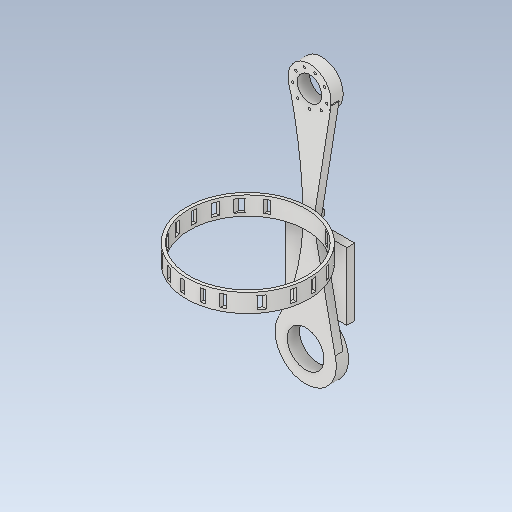
# Autodesk Inventor part: ES101_Project_Thigh support
Saved by Autodesk Inventor 2021 (Build 250183000, 183)
## iProperties
Created: 2021-03-10
Part Number: ES101_Project_Thigh support
Material: PPS Plastic
Document SubType Name: Modeling
Designer: lenovo
Density: 1.637 g/cm^3
Appearance: Smooth - White
Author: lenovo
Autodesk Inventor part; units mm, degrees
note: some values were not read from the file. Chosen so that the rebuilt part matches the saved one: second side of "Extrusion2"; second side of "Extrusion3".
ref_plane "YZ Plane" through (0, 0, 0) normal (1, 0, 0) x (0, 1, 0)
ref_plane "XY Plane" through (0, 0, 0) normal (0, 0, 1) x (1, 0, 0)
sketch "Sketch1" plane through (0, 0, 0) normal (0, 0, 1) x (1, 0, 0)
  arc A0 (-33.3712, 172.0844) -> (35.1489, 174.9362) centre (0.5971, 180.5198) ccw
  arc A1 (-50.7972, -166.0649) -> (-10.4253, -3.0182) centre (-368.5147, -0.8734) ccw
  line L0 (6.4335, -2.7585) -> (42.5482, -179.0984)
  arc A2 (42.5482, -179.0984) -> (-50.7972, -166.0649) centre (-6.4351, -189.1302) ccw
  arc A3 (-10.4253, -3.0182) -> (-33.3712, 172.0844) centre (-792.6654, -16.4703) ccw
  line L1 (6.4335, -2.7585) -> (35.1489, 174.9362)
  point P0 (0, 0)
  point P1 (-4.1446, -190.5357)
  point P2 (45.8554, -190.5357)
  dimension "d9" = 70
  dimension "d12" = 180
  dimension "d13" = 180
  dimension "d14" = 50
  constraints: 8 point on circle, 4 centre point, 4 end point, 4 tangent, 3 coincident
  measures "d9" diameter of A0
  measures "d12" distance of L0.start L0.end
  measures "d13" distance of L0.start L1.end
  measures "d14" radius of A2
extrude "Extrusion1" add sketch "Sketch1" along normal blind 13
sketch "Sketch2" plane through (0, 0, 13) normal (0, 0, 1) x (1, 0, 0)
  circle A0 centre (-6.3508, -188.8118) radius 50
  circle A1 centre (-6.3508, -188.8118) radius 30
  circle A2 centre (0, 180.6568) radius 35
  circle A3 centre (0, 180.6568) radius 20
  point P0 (0, 0)
  constraints: 4 centre point, 2 coincident
extrude "Extrusion2" add sketch "Sketch2" against normal blind 20 contours A0
sketch "Sketch3" plane through (0, 0, 13) normal (0, 0, 1) x (1, 0, 0)
  circle A0 centre (0, 182.0197) radius 35
  circle A1 centre (0, 182.0197) radius 20
  point P0 (0, 0)
  constraints: 2 centre point, 1 coincident
extrude "Extrusion3" add sketch "Sketch3" against normal blind 20
sketch "Sketch4" plane through (0, 0, 0) normal (0, 0, -1) x (-1, 0, 0)
  line L0 (-47.7429, -25.3634) -> (52.2571, -25.3634)
  line L1 (52.2571, -25.3634) -> (52.2571, -135.3634)
  line L2 (52.2571, -135.3634) -> (-47.7429, -135.3634)
  line L3 (-47.7429, -135.3634) -> (-47.7429, -25.3634)
  point P0 (0, 0)
  dimension "d32" = 100
  dimension "d33" = 110
  constraints: 8 end point, 2 parallel, 1 horizontal, 1 perpendicular
  measures "d32" distance of L1.end L2.end
  measures "d33" distance of L0.end L1.end
extrude "Extrusion4" add sketch "Sketch4" along normal blind 13
sketch "Sketch5" plane through (0, 0, 0) normal (0, 0, -1) x (-1, 0, 0)
  circle A0 centre (1.6929, -2.3398) radius 7
  point P0 (0, 0)
  constraints: 1 centre point
extrude "Extrusion5" add sketch "Sketch5" along normal blind 7
sketch "Sketch6" plane through (-1.6929, -2.3398, -7) normal (0, 0, -1) x (-1, 0, 0)
  circle A0 centre (0, 0) radius 7 projected
  circle A1 centre (0, 0) radius 5
  point P0 (-1.6929, 2.3398)
  dimension "d39" = 10
  constraints: 1 centre point, 1 coincident
  measures "d39" diameter of A1
extrude "Extrusion6" add sketch "Sketch6" along normal blind 2 contours A1
sketch "Sketch7" plane through (0, 0, 13) normal (0, 0, 1) x (1, 0, 0)
  point P0 (0, 0)
sketch "Sketch8" plane through (0, 0, 0) normal (0, 1, 0) x (-1, 0, 0)
  circle A0 centre (0, 113.7823) radius 100
  point P0 (0, 0)
  dimension "d88" = 200
  constraints: 1 centre point
  measures "d88" diameter of A0
extrude "Extrusion7" add sketch "Sketch8" along normal mid plane 30 separate body
sketch "Sketch9" plane through (0, 15, 113.7823) normal (0, 1, 0) x (1, 0, 0)
  circle A0 centre (0, 0) radius 95
  point P0 (0, 113.7823)
  dimension "d45" = 190
  constraints: 1 centre point
  measures "d45" diameter of A0
extrude "Extrusion8" cut sketch "Sketch9" against normal blind 30 bodies 2
sketch "Sketch10" plane through (0, 0, 13) normal (0, 0, 1) x (1, 0, 0)
  circle A0 centre (0, 177.9274) radius 34.5248
  point P0 (0, 0)
  constraints: 1 centre point
extrude "Extrusion9" add sketch "Sketch10" against normal blind 13 bodies 1
sketch "Sketch11" plane through (0, 182.0197, 0) normal (0, 0, -1) x (-1, 0, 0)
  circle A0 centre (0, 0) radius 20
  point P0 (0, -182.0197)
  constraints: 1 centre point
extrude "Extrusion10" cut sketch "Sketch11" against normal blind 13 bodies 1
sketch "Sketch12" plane through (0, 0, 13) normal (0, 0, 1) x (1, 0, 0)
  circle A0 centre (0, 153.4937) radius 2
  circle A1 centre (-19.2305, 158.9881) radius 2
  circle A2 centre (-27.7702, 177.0733) radius 2
  circle A3 centre (-22.2758, 196.3038) radius 2
  circle A4 centre (24.2555, 196.3038) radius 2
  circle A5 centre (28.2555, 175.0733) radius 2
  circle A6 centre (19.1953, 160.9881) radius 2
  circle A7 centre (-8.7701, 208.0286) radius 2
  circle A8 centre (9.0493, 208.0286) radius 2
  point P0 (0, 0)
  dimension "d54" = 4
  dimension "d67" = 4
  dimension "d68" = 4
  dimension "d69" = 4
  constraints: 9 centre point
  measures "d54" diameter of A0
  measures "d67" diameter of A6
  measures "d68" diameter of A7
  measures "d69" diameter of A8
extrude "Extrusion11" cut sketch "Sketch12" against normal blind 20 bodies 1
sketch "Sketch13" plane through (0, 0, 0) normal (1, 0, 0) x (0, 1, 0)
  point P0 (0, 0)
sketch "Sketch14" plane through (0, 0, 13) normal (0, 0, 1) x (1, 0, 0)
  point P0 (0, 0)
sketch "Sketch15" plane through (0, 0, 0) normal (1, 0, 0) x (0, 1, 0)
  point P0 (0, 0)
ref_plane "Work Plane1" through (0, 0, 0) normal (0, 1, 0) x (-1, 0, 0)
sketch "Sketch16" plane through (0, 0, 0) normal (0, 1, 0) x (-1, 0, 0)
  line L0 (32.5367, 18.2576) -> (29.6883, 18.2576)
  line L1 (29.6883, 18.2576) -> (29.6883, 28.4518)
  line L2 (29.6883, 28.4518) -> (32.5367, 28.4518)
  line L3 (32.5367, 28.4518) -> (32.5367, 18.2576)
  line L4 (12.3378, 34.8063) -> (36.3483, 52.7924)
  line L5 (36.3483, 52.7924) -> (49.6954, 79.6597)
  line L6 (49.6954, 79.6597) -> (51.0134, 109.6307)
  line L7 (51.0134, 109.6307) -> (41.4291, 138.0586)
  line L8 (41.4291, 138.0586) -> (20.4475, 159.5009)
  line L9 (20.4475, 159.5009) -> (-7.3084, 170.8857)
  line L10 (-7.3084, 170.8857) -> (-37.3084, 170.8857)
  line L11 (-37.3084, 170.8857) -> (-63.9806, 157.1528)
  line L12 (-63.9806, 157.1528) -> (-83.8606, 134.6853)
  line L13 (-83.8606, 134.6853) -> (-92.5467, 105.9703)
  line L14 (-92.5467, 105.9703) -> (-89.9607, 76.082)
  line L15 (-89.9607, 76.082) -> (-73.9206, 50.7302)
  line L16 (-73.9206, 50.7302) -> (-48.4956, 34.8063)
  line L17 (38.6924, 42.1786) -> (34.0041, 42.1786)
  line L18 (34.0041, 42.1786) -> (34.0041, 63.4061)
  line L19 (34.0041, 63.4061) -> (38.6924, 63.4061)
  line L20 (38.6924, 63.4061) -> (38.6924, 42.1786)
  line L21 (38.6924, 42.1786) -> (34.0041, 63.4061) construction
  line L22 (34.0041, 42.1786) -> (38.6924, 63.4061) construction
  line L23 (53.1695, 77.9338) -> (46.2212, 77.9338)
  line L24 (46.2212, 77.9338) -> (46.2212, 81.3856)
  line L25 (46.2212, 81.3856) -> (53.1695, 81.3856)
  line L26 (53.1695, 81.3856) -> (53.1695, 77.9338)
  line L27 (53.1695, 77.9338) -> (46.2212, 81.3856) construction
  line L28 (46.2212, 77.9338) -> (53.1695, 81.3856) construction
  line L29 (55.8056, 106.9834) -> (46.2212, 106.9834)
  line L30 (46.2212, 106.9834) -> (46.2212, 112.2781)
  line L31 (46.2212, 112.2781) -> (55.8056, 112.2781)
  line L32 (55.8056, 112.2781) -> (55.8056, 106.9834)
  line L33 (55.8056, 106.9834) -> (46.2212, 112.2781) construction
  line L34 (46.2212, 106.9834) -> (55.8056, 112.2781) construction
  line L35 (49.7019, 140.8477) -> (33.1562, 140.8477)
  line L36 (33.1562, 140.8477) -> (33.1562, 135.2694)
  line L37 (33.1562, 135.2694) -> (49.7019, 135.2694)
  line L38 (49.7019, 135.2694) -> (49.7019, 140.8477)
  line L39 (49.7019, 140.8477) -> (33.1562, 135.2694) construction
  line L40 (33.1562, 140.8477) -> (49.7019, 135.2694) construction
  line L41 (23.199, 166.209) -> (17.696, 166.209)
  line L42 (17.696, 166.209) -> (17.696, 152.7928)
  line L43 (17.696, 152.7928) -> (23.199, 152.7928)
  line L44 (23.199, 152.7928) -> (23.199, 166.209)
  line L45 (23.199, 166.209) -> (17.696, 152.7928) construction
  line L46 (17.696, 166.209) -> (23.199, 152.7928) construction
  line L47 (-4.671, 165.1258) -> (-9.9457, 165.1258)
  line L48 (-9.9457, 165.1258) -> (-9.9457, 176.6455)
  line L49 (-9.9457, 176.6455) -> (-4.671, 176.6455)
  line L50 (-4.671, 176.6455) -> (-4.671, 165.1258)
  line L51 (-4.671, 165.1258) -> (-9.9457, 176.6455) construction
  line L52 (-9.9457, 165.1258) -> (-4.671, 176.6455) construction
  line L53 (-34.1603, 165.1258) -> (-40.4564, 165.1258)
  line L54 (-40.4564, 165.1258) -> (-40.4564, 176.6455)
  line L55 (-40.4564, 176.6455) -> (-34.1603, 176.6455)
  line L56 (-34.1603, 176.6455) -> (-34.1603, 165.1258)
  line L57 (-34.1603, 165.1258) -> (-40.4564, 176.6455) construction
  line L58 (-40.4564, 165.1258) -> (-34.1603, 176.6455) construction
  line L59 (-61.4196, 149.1797) -> (-66.5415, 149.1797)
  line L60 (-66.5415, 149.1797) -> (-66.5415, 165.1258)
  line L61 (-66.5415, 165.1258) -> (-61.4196, 165.1258)
  line L62 (-61.4196, 165.1258) -> (-61.4196, 149.1797)
  line L63 (-61.4196, 149.1797) -> (-66.5415, 165.1258) construction
  line L64 (-66.5415, 149.1797) -> (-61.4196, 165.1258) construction
  line L65 (-77.7604, 131.3121) -> (-89.9607, 131.3121)
  line L66 (-89.9607, 131.3121) -> (-89.9607, 138.0586)
  line L67 (-89.9607, 138.0586) -> (-77.7604, 138.0586)
  line L68 (-77.7604, 138.0586) -> (-77.7604, 131.3121)
  line L69 (-77.7604, 131.3121) -> (-89.9607, 138.0586) construction
  line L70 (-89.9607, 131.3121) -> (-77.7604, 138.0586) construction
  line L71 (-83.9584, 102.3099) -> (-101.135, 102.3099)
  line L72 (-101.135, 102.3099) -> (-101.135, 109.6307)
  line L73 (-101.135, 109.6307) -> (-83.9584, 109.6307)
  line L74 (-83.9584, 109.6307) -> (-83.9584, 102.3099)
  line L75 (-83.9584, 102.3099) -> (-101.135, 109.6307) construction
  line L76 (-101.135, 102.3099) -> (-83.9584, 109.6307) construction
  line L77 (-81.3841, 74.2301) -> (-98.5373, 74.2301)
  line L78 (-98.5373, 74.2301) -> (-98.5373, 77.9338)
  line L79 (-98.5373, 77.9338) -> (-81.3841, 77.9338)
  line L80 (-81.3841, 77.9338) -> (-81.3841, 74.2301)
  line L81 (-81.3841, 74.2301) -> (-98.5373, 77.9338) construction
  line L82 (-98.5373, 74.2301) -> (-81.3841, 77.9338) construction
  circle A0 centre (0, 113.7823) radius 95 projected
  line L83 (-70.6836, 43.1011) -> (-77.1576, 43.1011)
  line L84 (-77.1576, 43.1011) -> (-77.1576, 58.3593)
  line L85 (-77.1576, 58.3593) -> (-70.6836, 58.3593)
  line L86 (-70.6836, 58.3593) -> (-70.6836, 43.1011)
  line L87 (-70.6836, 43.1011) -> (-77.1576, 58.3593) construction
  line L88 (-77.1576, 43.1011) -> (-70.6836, 58.3593) construction
  point P0 (0, 0)
  point P1 (20.4475, 159.5009)
  point P2 (-83.8606, 134.6853)
  point P3 (-92.5467, 105.9703)
  point P4 (-31.8698, 21.1136)
  dimension "d73" = 30
  dimension "d74" = 30
  dimension "d75" = 30
  dimension "d76" = 30
  dimension "d77" = 30
  dimension "d78" = 30
  dimension "d79" = 30
  dimension "d80" = 30
  dimension "d81" = 30
  dimension "d82" = 30
  dimension "d83" = 30
  dimension "d84" = 30
  dimension "d85" = 30
  constraints: 178 end point, 26 parallel, 24 midpoint, 14 horizontal, 13 coincident, 13 perpendicular, 4 point on line, 2 other
  measures "d73" distance of L4.start L4.end
  measures "d74" distance of L4.end L5.end
  measures "d75" distance of L5.end L6.end
  measures "d76" distance of L6.end L7.end
  measures "d77" distance of L7.end L8.end
  measures "d78" distance of L8.end L9.end
  measures "d79" distance of L9.end L10.end
  measures "d80" distance of L10.end L11.end
  measures "d81" distance of L11.end L12.end
  measures "d82" distance of L12.end L13.end
  measures "d83" distance of L13.end L14.end
  measures "d84" distance of L14.end L15.end
  measures "d85" distance of L15.end L16.end
extrude "Extrusion12" cut sketch "Sketch16" along normal mid plane 20 contours A0 L71 L72 L73 | L73 L13 L14 L71 A0 | L86 L83 L84 L15 L16 | L16 L15 L84 A0 L86 | A0 L85 L86 | L73 L74 L71 L14 L13 | A0 L79 L80 L77 | L77 L15 L14 L79 A0 | L14 L15 L77 L78 L79 | L18 L19 L20 L5 L4 | L4 L5 L20 L17 L18 | L23 L24 L25 L6 L5 | L5 L6 L25 L26 L23 | L29 L30 L31 L7 L6 | L6 L7 L31 L32 L29 | L37 L36 L35 L8 L7 | L7 L8 L35 L38 L37 | L44 L43 L42 L9 L8 | L8 L9 L42 L41 L44 | L50 L47 L48 L10 L9 | L9 L10 L48 L49 L50 | L56 L53 L54 L11 L10 | L10 L11 L54 L55 L56 | L62 L59 L60 L12 L11 | L11 L12 L60 L61 L62 | L67 L68 L65 L13 L12 | L12 L13 L65 L66 L67 bodies 2
sketch "Sketch17" plane through (0, 0, 0) normal (0, 1, 0) x (-1, 0, 0)
  point P0 (0, 0)
sketch "Sketch18" plane through (0, 0, 0) normal (0, 1, 0) x (-1, 0, 0)
  point P0 (0, 0)
sketch "Sketch19" plane through (0, 0, 0) normal (0, 1, 0) x (-1, 0, 0)
  circle A0 centre (0, 113.7823) radius 95 projected
  line L0 (52.8651, 18.7823) -> (45.8007, 18.7823)
  line L1 (45.8007, 18.7823) -> (45.8007, 41.1386)
  line L2 (45.8007, 41.1386) -> (52.8651, 41.1386)
  line L3 (52.8651, 41.1386) -> (52.8651, 18.7823)
  line L4 (77.5737, 41.1386) -> (69.4706, 41.1386)
  line L5 (69.4706, 41.1386) -> (69.4706, 64.2531)
  line L6 (69.4706, 64.2531) -> (77.5737, 64.2531)
  line L7 (77.5737, 64.2531) -> (77.5737, 41.1386)
  line L8 (98.2601, 73.8776) -> (86.2126, 73.8776)
  line L9 (86.2126, 73.8776) -> (86.2126, 82.7453)
  line L10 (86.2126, 82.7453) -> (98.2601, 82.7453)
  line L11 (98.2601, 82.7453) -> (98.2601, 73.8776)
  line L12 (100, 102.7509) -> (92.2364, 102.7509)
  line L13 (92.2364, 102.7509) -> (92.2364, 110.3271)
  line L14 (92.2364, 110.3271) -> (100, 110.3271)
  line L15 (100, 110.3271) -> (100, 102.7509)
  line L16 (104.0063, 132.7242) -> (86.2126, 132.7242)
  line L17 (86.2126, 132.7242) -> (86.2126, 140.2074)
  line L18 (86.2126, 140.2074) -> (104.0063, 140.2074)
  line L19 (104.0063, 140.2074) -> (104.0063, 132.7242)
  line L20 (92.2364, 160.8086) -> (69.4706, 160.8086)
  line L21 (69.4706, 160.8086) -> (69.4706, 167.7891)
  line L22 (69.4706, 167.7891) -> (92.2364, 167.7891)
  line L23 (92.2364, 167.7891) -> (92.2364, 160.8086)
  line L24 (63.7642, 176.4983) -> (56.8874, 176.4983)
  line L25 (56.8874, 176.4983) -> (56.8874, 200.5755)
  line L26 (56.8874, 200.5755) -> (63.7642, 200.5755)
  line L27 (63.7642, 200.5755) -> (63.7642, 176.4983)
  line L28 (38.6255, 188.5369) -> (31.0295, 188.5369)
  line L29 (31.0295, 188.5369) -> (31.0295, 217.7811)
  line L30 (31.0295, 217.7811) -> (38.6255, 217.7811)
  line L31 (38.6255, 217.7811) -> (38.6255, 188.5369)
  line L32 (9.635, 195.622) -> (3.4477, 195.622)
  line L33 (3.4477, 195.622) -> (3.4477, 223.5273)
  line L34 (3.4477, 223.5273) -> (9.635, 223.5273)
  line L35 (9.635, 223.5273) -> (9.635, 195.622)
  line L36 (-20.3163, 195.622) -> (-27.5818, 195.622)
  line L37 (-27.5818, 195.622) -> (-27.5818, 223.5273)
  line L38 (-27.5818, 223.5273) -> (-20.3163, 223.5273)
  line L39 (-20.3163, 223.5273) -> (-20.3163, 195.622)
  line L40 (-44.2729, 188.5369) -> (-51.1235, 188.5369)
  line L41 (-51.1235, 188.5369) -> (-51.1235, 217.7811)
  line L42 (-51.1235, 217.7811) -> (-44.2729, 217.7811)
  line L43 (-44.2729, 217.7811) -> (-44.2729, 188.5369)
  line L44 (-63.2776, 167.7891) -> (-87.3549, 167.7891)
  line L45 (-87.3549, 167.7891) -> (-87.3549, 176.4983)
  line L46 (-87.3549, 176.4983) -> (-63.2776, 176.4983)
  line L47 (-63.2776, 176.4983) -> (-63.2776, 167.7891)
  line L48 (-82.4014, 132.7242) -> (-108.1813, 132.7242)
  line L49 (-108.1813, 132.7242) -> (-108.1813, 140.2074)
  line L50 (-108.1813, 140.2074) -> (-82.4014, 140.2074)
  line L51 (-82.4014, 140.2074) -> (-82.4014, 132.7242)
  line L52 (-40.7376, 15.6418) -> (-47.6982, 15.6418)
  line L53 (-47.6982, 15.6418) -> (-47.6982, 45.1304)
  line L54 (-47.6982, 45.1304) -> (-40.7376, 45.1304)
  line L55 (-40.7376, 45.1304) -> (-40.7376, 15.6418)
  point P0 (0, 0)
  point P1 (45.8007, 30.5519)
  point P2 (69.4706, 48.9838)
  point P3 (94.3573, 102.7509)
  point P4 (93.0924, 132.7242)
  point P5 (82.5441, 160.8086)
  point P6 (63.7642, 184.2033)
  point P7 (38.6255, 200.5755)
  point P8 (9.635, 208.2924)
  point P9 (-20.3163, 206.5845)
  point P10 (-48.2416, 195.622)
  point P11 (-71.3562, 176.4983)
  point P12 (-87.3549, 151.1203)
  point P13 (-95.0718, 122.1298)
  point P14 (-93.3638, 92.1784)
  point P15 (-82.4014, 64.2531)
  point P16 (-63.2776, 41.1386)
  point P17 (-37.8996, 25.1399)
  constraints: 112 end point, 28 parallel, 14 horizontal, 14 perpendicular, 6 point on line
extrude "Extrusion13" cut sketch "Sketch19" along normal mid plane 20 bodies 2
body "Solid1"
body "Solid2"
